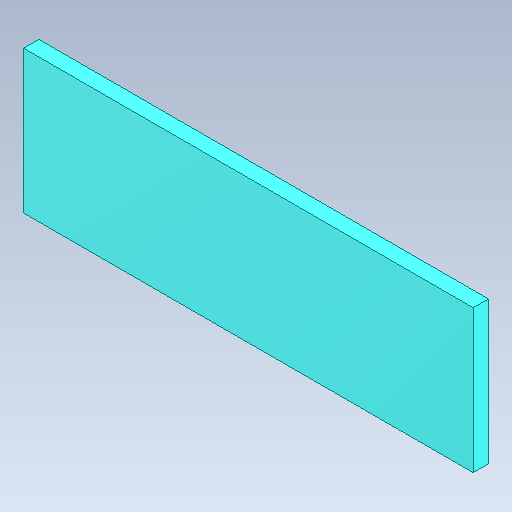
# Autodesk Inventor part: VTA52
Saved by Autodesk Inventor 2021 (Build 250183000, 183)
## iProperties
Created: 2020-11-18
Part Number: VTA52
Material: Generic
Document SubType Name: Modeling
Designer: Admin
Density: 1 g/cm^3
Appearance: VTA52, VTA52
Author: Admin
Autodesk Inventor part; units mm, degrees
ref_plane "YZ Plane" through (0, 0, 0) normal (1, 0, 0) x (0, 1, 0)
ref_plane "XZ Plane" through (0, 0, 0) normal (0, 1, 0) x (-1, 0, 0)
ref_plane "XY Plane" through (0, 0, 0) normal (0, 0, 1) x (1, 0, 0)
sketch "VTA52, VTA52_36" plane through (0, 0, 0) normal (0, 0, 1) x (1, 0, 0)
  line L0 (-15.5448, 4.725) -> (13.97, 4.725)
  line L1 (13.97, 4.725) -> (13.97, -4.65)
  line L2 (13.97, -4.65) -> (-15.5448, -4.65)
  line L3 (-15.5448, -4.65) -> (-15.5448, 4.725)
  constraints: 8 end point
extrude "Extrusion1" add sketch "VTA52, VTA52_36" along normal blind 1
body "Solid1"
